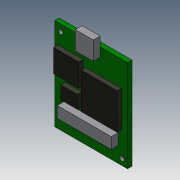
# Autodesk Inventor part: NEUROPIXEL HEADSTAGE PCB
Saved by Autodesk Inventor 2018.3 (Build 223284000, 284)
## iProperties
Created: 2017-08-07
Material: Generic
Vendor: IMEC
Document SubType Name: Modeling
Designer: ARNOLDJ
Density: 1 g/cm^3
Appearance: Default
Description: NEUROPIXEL HEADSTAGE PCB
RuleStatus: InUse
AfterDocSave0: file://Part Number Cleaner
DESIGN DEPARTMENT: HHMI: JRC - ID&F
ALTERED ITEM PART NUMBER: N/A
ALTERED ITEM VENDOR: N/A
ALTERED ITEM DESCRIPTION: N/A
Author: ARNOLDJ
Revision Number: 0
Autodesk Inventor part; units mm, degrees
ref_plane "YZ Plane" through (0, 0, 0) normal (1, 0, 0) x (0, 1, 0)
ref_plane "XZ Plane" through (0, 0, 0) normal (0, 1, 0) x (-1, 0, 0)
ref_plane "XY Plane" through (0, 0, 0) normal (0, 0, 1) x (1, 0, 0)
sketch "Sketch1" plane through (0, 0, 0) normal (0, 0, 1) x (1, 0, 0)
  line L0 (0, 133.1936) -> (0, -174.4071) projected
  line L1 (-87.3177, 0) -> (127.2932, 0) projected
  line L2 (8, -10.1) -> (-8, -10.1)
  line L3 (-8, -10.1) -> (-8, 10.1)
  line L4 (-8, 10.1) -> (8, 10.1)
  line L5 (8, 10.1) -> (8, -10.1)
  line L6 (8, -10.1) -> (-8, 10.1) construction
  line L7 (-8, -10.1) -> (8, 10.1) construction
  circle A0 centre (-6.731, 8.636) radius 0.5139 construction
  circle A1 centre (6.731, -8.763) radius 0.49 construction
  line L8 (-5.9376, -4.2616) -> (5.9143, -4.2616)
  line L9 (5.9143, -4.2616) -> (5.9143, -6.7235)
  line L10 (5.9143, -6.7235) -> (-5.9376, -6.7235)
  line L11 (-5.9376, -6.7235) -> (-5.9376, -4.2616)
  line L12 (-1.9876, 12.1457) -> (1.9674, 12.1457)
  line L13 (1.9674, 12.1457) -> (1.9674, 8.0874)
  line L14 (1.9674, 8.0874) -> (-1.9876, 8.0874)
  line L15 (-1.9876, 8.0874) -> (-1.9876, 12.1457)
  line L16 (-7.2449, 5.8703) -> (-1.7339, 5.8703)
  line L17 (-1.7339, 5.8703) -> (-1.7339, 0.8708)
  line L18 (-1.7339, 0.8708) -> (-7.2449, 0.8708)
  line L19 (-7.2449, 0.8708) -> (-7.2449, 5.8703)
  line L20 (-5.683, -0.4539) -> (-1.9876, -0.4539)
  line L21 (-1.9876, -0.4539) -> (-1.9876, -3.3033)
  line L22 (-1.9876, -3.3033) -> (-5.683, -3.3033)
  line L23 (-5.683, -3.3033) -> (-5.683, -0.4539)
  line L24 (-1.184, 4.5949) -> (6.731, 4.5949)
  line L25 (6.731, 4.5949) -> (6.731, -3.3033)
  line L26 (6.731, -3.3033) -> (-1.184, -3.3033)
  line L27 (-1.184, -3.3033) -> (-1.184, 4.5949)
  line L28 (54.8091, 13.2903) -> (96.6345, 13.2903) construction
  line L29 (96.6345, 13.2903) -> (96.6345, -86.1085) construction
  line L30 (96.6345, -86.1085) -> (54.8091, -86.1085) construction
  line L31 (54.8091, -86.1085) -> (54.8091, 13.2903) construction
  line L32 (-7.642, -75.3683) -> (-7.642, -85.3683)
  line L33 (71.1512, 85.7776) -> (64.977, -130.4641) construction
  line L34 (64.977, -130.4641) -> (-56.659, -126.9911) construction
  line L35 (-56.659, -126.9911) -> (-50.4848, 89.2506) construction
  line L36 (-50.4848, 89.2506) -> (71.1512, 85.7776) construction
  point P0 (0, 0)
  dimension "d0" = 16
  dimension "d54" = 20.2
  dimension "d67" = 8.636
  dimension "d68" = 6.731
  dimension "d69" = 8.763
  dimension "d70" = 6.731
  dimension "d173" = 17.399
  dimension "d175" = 10
  dimension "d232" = 13.462
  constraints: 54 end point, 12 parallel, 6 horizontal, 6 perpendicular, 2 centre point, 2 coincident, 2 midpoint, 1 point on line, 1 vertical, 4 other
  measures "d0" distance of L3.end L4.end
  measures "d54" distance of L2.end L3.end
  measures "d67" distance from line of L1 point (-6.731, 8.636)
  measures "d68" distance from line of L0 point (-6.731, 8.636)
  measures "d69" distance from line of point (6.731, -8.763) L1
  measures "d70" distance from line of point (6.731, -8.763) L0
  measures "d173" vertical distance of A1.centre A0.centre
  measures "d175" distance of L32.start L32.end
  measures "d232" horizontal distance of A1.centre A0.centre
extrude "Extrusion1" add sketch "Sketch1" against normal blind 1 contours L4 L13 L14 L0 | L0 L14 L15 L4 | L14 L13 L4 L5 L1 L25 L24 L0 | L0 L24 L27 L1 L3 L4 L15 L14 | L24 L25 L1 L0 | L0 L1 L27 L24 | L1 L25 L26 L0 | L0 L26 L27 L1 | L1 L27 L26 L0 L8 L11 L10 L2 L3 | L5 L2 L0 L10 L9 L8 L26 L25 L1 | L8 L9 L10 L0 | L0 L10 L11 L8 | L16 L17 L18 L19 | L20 L21 L22 L23
extrude "Extrusion2" add sketch "Sketch1" along normal blind 1 contours L24 L25 L1 L0 | L0 L1 L27 L24 | L1 L25 L26 L0 | L0 L26 L27 L1 | L16 L17 L18 L19 | L20 L21 L22 L23
extrude "Extrusion3" add sketch "Sketch1" along normal blind 1.5 contours L12 L13 L4 L0 | L0 L4 L15 L12 | L4 L13 L14 L0 | L0 L14 L15 L4 | L8 L9 L10 L0 | L0 L10 L11 L8
hole "Hole1" at (6.731, -8.763, 0) at (-6.731, 8.636, 0) direction (0, 0, -1) diameter 1 depth 25.4 tip angle 118
body "Solid1"
